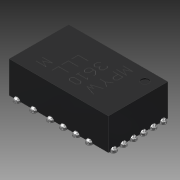
# Autodesk Inventor part: MPM3610 Step-Down Module
Saved by Autodesk Inventor 2016 (Build 200138000, 138)
## iProperties
Created: 2019-08-17
Part Number: MPM3610 Step-Down Module
Material: Generic
Document SubType Name: Modeling
Designer: Orest
Mass: 0.0242835 g
Surface Area: 0.598221 cm^2
Volume: 0.0242835 cm^3
Density: 1 g/cm^3
Appearance: Smooth - Black (BGA)
Author: Orest
Autodesk Inventor part; units mm, degrees
ref_plane "YZ Plane" through (0, 0, 0) normal (1, 0, 0) x (0, 1, 0)
ref_plane "XZ Plane" through (0, 0, 0) normal (0, 1, 0) x (-1, 0, 0)
sketch "Sketch10" plane through (0, 0, 0) normal (0, 1, 0) x (-1, 0, 0)
  line L0 (-1.5, -2.5) -> (1.5, -2.5)
  line L1 (1.5, -2.5) -> (1.5, 2.5)
  line L2 (1.5, 2.5) -> (-1.5, 2.5)
  line L3 (-1.5, 2.5) -> (-1.5, -2.5)
  line L4 (-1.5, -2.5) -> (1.5, 2.5) construction
  line L5 (1.5, -2.5) -> (-1.5, 2.5) construction
  point P0 (0, 0)
  point P1 (0, 0)
  dimension "d7" = 3
  dimension "d8" = 5
  constraints: 12 end point, 2 parallel, 1 coincident, 1 horizontal, 1 midpoint, 1 perpendicular
  measures "d7" distance of L1.end L2.end
  measures "d8" distance of L0.end L1.end
extrude "Extrusion4" add sketch "Sketch10" along normal mid plane 1.6
sketch "Sketch11" plane through (0, 0.8, 0) normal (0, 1, 0) x (1, 0, 0)
  circle A0 centre (0.95, -1.9) radius 0.2
  line L0 (1.5, 2.5) -> (-1.5, 2.5) construction
  line L1 (-1.5, 2.5) -> (-1.5, -2.5) construction
  line L2 (-1.5, -2.5) -> (1.5, -2.5) construction
  line L3 (1.5, -2.5) -> (1.5, 2.5) construction
  line L4 (1, -1.55) -> (-1, -1.55) construction
  line L5 (-1, -1.55) -> (-1, 2.1) construction
  line L6 (-1, 2.1) -> (1, 2.1) construction
  line L7 (1, 2.1) -> (1, -1.55) construction
  line L8 (0.7272, -0.6725) -> (0.7519, -0.6725)
  line L9 (0.7519, -0.6725) -> (0.7519, -1.1357)
  line L10 (0.7519, -1.1357) -> (0.9018, -0.8225)
  line L11 (0.9018, -0.8225) -> (1.0514, -1.1357)
  line L12 (1.0514, -1.1357) -> (1.0514, -0.6725)
  line L13 (1.0514, -0.6725) -> (1.076, -0.6725)
  line L14 (1.076, -0.6725) -> (1.076, -1.1725)
  line L15 (1.076, -1.1725) -> (1.0535, -1.1725)
  line L16 (1.0535, -1.1725) -> (0.9018, -0.8605)
  line L17 (0.9018, -0.8605) -> (0.7502, -1.1725)
  line L18 (0.7502, -1.1725) -> (0.7272, -1.1725)
  line L19 (0.7272, -1.1725) -> (0.7272, -0.6725)
  line L20 (0.2306, -0.9987) -> (0.3191, -0.9102)
  line L21 (0.3191, -0.9102) -> (0.5547, -0.9102)
  line L22 (0.5547, -0.9102) -> (0.5547, -0.6725)
  line L23 (0.5547, -0.6725) -> (0.5794, -0.6725)
  line L24 (0.5794, -0.6725) -> (0.5794, -1.1775)
  line L25 (0.5794, -1.1775) -> (0.3191, -1.1775)
  line L26 (0.3191, -1.1775) -> (0.2306, -1.089)
  line L27 (0.2306, -1.089) -> (0.2306, -0.9987)
  line L28 (0.2552, -1.0083) -> (0.2552, -1.0798)
  line L29 (0.2552, -1.0798) -> (0.3296, -1.1537)
  line L30 (0.3296, -1.1537) -> (0.5547, -1.1537)
  line L31 (0.5547, -1.1537) -> (0.5547, -0.9344)
  line L32 (0.5547, -0.9344) -> (0.3292, -0.9344)
  line L33 (0.3292, -0.9344) -> (0.2552, -1.0083)
  line L34 (-0.2652, -1.1654) -> (-0.1036, -0.9194)
  line L35 (-0.1036, -0.9194) -> (-0.1036, -0.6725)
  line L36 (-0.1036, -0.6725) -> (-0.0789, -0.6725)
  line L37 (-0.0789, -0.6725) -> (-0.0789, -0.9189)
  line L38 (-0.0789, -0.9189) -> (0.0823, -1.1654)
  line L39 (0.0823, -1.1654) -> (0.0639, -1.175)
  line L40 (0.0639, -1.175) -> (-0.0915, -0.9386)
  line L41 (-0.0915, -0.9386) -> (-0.2464, -1.175)
  line L42 (-0.2464, -1.175) -> (-0.2652, -1.1654)
  line L43 (-0.9244, -1.1675) -> (-0.7607, -0.6725)
  line L44 (-0.7607, -0.6725) -> (-0.7393, -0.6725)
  line L45 (-0.7393, -0.6725) -> (-0.6692, -0.8989)
  line L46 (-0.6692, -0.8989) -> (-0.5986, -0.6725)
  line L47 (-0.5986, -0.6725) -> (-0.5777, -0.6725)
  line L48 (-0.5777, -0.6725) -> (-0.414, -1.1675)
  line L49 (-0.414, -1.1675) -> (-0.4357, -1.1742)
  line L50 (-0.4357, -1.1742) -> (-0.5881, -0.703)
  line L51 (-0.5881, -0.703) -> (-0.6688, -0.9461)
  line L52 (-0.6688, -0.9461) -> (-0.7502, -0.703)
  line L53 (-0.7502, -0.703) -> (-0.9023, -1.1742)
  line L54 (-0.9023, -1.1742) -> (-0.9244, -1.1675)
  line L55 (0.3137, 0.0444) -> (0.4023, 0.1325)
  line L56 (0.4023, 0.1325) -> (0.5744, 0.1325)
  line L57 (0.5744, 0.1325) -> (0.6612, 0.0435)
  line L58 (0.6612, 0.0435) -> (0.6466, 0.0289)
  line L59 (0.6466, 0.0289) -> (0.5647, 0.1087)
  line L60 (0.5647, 0.1087) -> (0.4123, 0.1087)
  line L61 (0.4123, 0.1087) -> (0.3383, 0.0348)
  line L62 (0.3383, 0.0348) -> (0.3383, -0.0367)
  line L63 (0.3383, -0.0367) -> (0.4127, -0.1102)
  line L64 (0.4127, -0.1102) -> (0.495, -0.1102)
  line L65 (0.495, -0.1102) -> (0.495, -0.1344)
  line L66 (0.495, -0.1344) -> (0.4123, -0.1344)
  line L67 (0.4123, -0.1344) -> (0.3383, -0.2083)
  line L68 (0.3383, -0.2083) -> (0.3383, -0.2793)
  line L69 (0.3383, -0.2793) -> (0.4127, -0.3537)
  line L70 (0.4127, -0.3537) -> (0.5643, -0.3537)
  line L71 (0.5643, -0.3537) -> (0.6466, -0.2739)
  line L72 (0.6466, -0.2739) -> (0.6612, -0.2885)
  line L73 (0.6612, -0.2885) -> (0.5744, -0.3775)
  line L74 (0.5744, -0.3775) -> (0.4023, -0.3775)
  line L75 (0.4023, -0.3775) -> (0.3137, -0.289)
  line L76 (0.3137, -0.289) -> (0.3137, -0.1987)
  line L77 (0.3137, -0.1987) -> (0.3931, -0.1223)
  line L78 (0.3931, -0.1223) -> (0.3137, -0.0458)
  line L79 (0.3137, -0.0458) -> (0.3137, 0.0444)
  line L80 (-0.183, 0.0444) -> (-0.0944, 0.1325)
  line L81 (-0.0944, 0.1325) -> (0.0777, 0.1325)
  line L82 (0.0777, 0.1325) -> (0.1658, 0.0448)
  line L83 (0.1658, 0.0448) -> (0.1658, -0.2083)
  line L84 (0.1658, -0.2083) -> (-0.0033, -0.3775)
  line L85 (-0.0033, -0.3775) -> (-0.0961, -0.3775)
  line L86 (-0.0961, -0.3775) -> (-0.0961, -0.3537)
  line L87 (-0.0961, -0.3537) -> (-0.0134, -0.3537)
  line L88 (-0.0134, -0.3537) -> (0.1412, -0.1987)
  line L89 (0.1412, -0.1987) -> (0.1412, -0.1344)
  line L90 (0.1412, -0.1344) -> (-0.0944, -0.1344)
  line L91 (-0.0944, -0.1344) -> (-0.183, -0.0458)
  line L92 (-0.183, -0.0458) -> (-0.183, 0.0444)
  line L93 (-0.1583, 0.0348) -> (-0.1583, -0.0367)
  line L94 (-0.1583, -0.0367) -> (-0.084, -0.1102)
  line L95 (-0.084, -0.1102) -> (0.1412, -0.1102)
  line L96 (0.1412, -0.1102) -> (0.1412, 0.0352)
  line L97 (0.1412, 0.0352) -> (0.0681, 0.1087)
  line L98 (0.0681, 0.1087) -> (-0.0844, 0.1087)
  line L99 (-0.0844, 0.1087) -> (-0.1583, 0.0348)
  line L100 (-0.5121, 0.1325) -> (-0.3358, 0.1325)
  line L101 (-0.3358, 0.1325) -> (-0.3358, 0.1087)
  line L102 (-0.3358, 0.1087) -> (-0.4119, 0.1087)
  line L103 (-0.4119, 0.1087) -> (-0.4119, -0.3462)
  line L104 (-0.4119, -0.3462) -> (-0.3467, -0.2739)
  line L105 (-0.3467, -0.2739) -> (-0.3321, -0.2885)
  line L106 (-0.3321, -0.2885) -> (-0.4185, -0.3775)
  line L107 (-0.4185, -0.3775) -> (-0.4361, -0.3775)
  line L108 (-0.4361, -0.3775) -> (-0.4361, 0.1087)
  line L109 (-0.4361, 0.1087) -> (-0.5121, 0.1087)
  line L110 (-0.5121, 0.1087) -> (-0.5121, 0.1325)
  line L111 (-0.9298, 0.0444) -> (-0.8413, 0.1325)
  line L112 (-0.8413, 0.1325) -> (-0.7502, 0.1325)
  line L113 (-0.7502, 0.1325) -> (-0.6621, 0.0448)
  line L114 (-0.6621, 0.0448) -> (-0.6621, -0.2894)
  line L115 (-0.6621, -0.2894) -> (-0.7502, -0.3775)
  line L116 (-0.7502, -0.3775) -> (-0.8413, -0.3775)
  line L117 (-0.8413, -0.3775) -> (-0.9298, -0.289)
  line L118 (-0.9298, -0.289) -> (-0.9298, 0.0444)
  line L119 (-0.9052, 0.0348) -> (-0.9052, -0.2798)
  line L120 (-0.9052, -0.2798) -> (-0.8312, -0.3537)
  line L121 (-0.8312, -0.3537) -> (-0.7602, -0.3537)
  line L122 (-0.7602, -0.3537) -> (-0.6867, -0.2798)
  line L123 (-0.6867, -0.2798) -> (-0.6867, 0.0352)
  line L124 (-0.6867, 0.0352) -> (-0.7598, 0.1087)
  line L125 (-0.7598, 0.1087) -> (-0.8312, 0.1087)
  line L126 (-0.8312, 0.1087) -> (-0.9052, 0.0348)
  line L127 (0.071, 0.9325) -> (0.414, 0.9325)
  line L128 (0.414, 0.9325) -> (0.414, 0.4275)
  line L129 (0.414, 0.4275) -> (0.3893, 0.4275)
  line L130 (0.3893, 0.4275) -> (0.3893, 0.9087)
  line L131 (0.3893, 0.9087) -> (0.071, 0.9087)
  line L132 (0.071, 0.9087) -> (0.071, 0.9325)
  line L133 (-0.4256, 0.9325) -> (-0.0827, 0.9325)
  line L134 (-0.0827, 0.9325) -> (-0.0827, 0.4275)
  line L135 (-0.0827, 0.4275) -> (-0.1074, 0.4275)
  line L136 (-0.1074, 0.4275) -> (-0.1074, 0.9087)
  line L137 (-0.1074, 0.9087) -> (-0.4256, 0.9087)
  line L138 (-0.4256, 0.9087) -> (-0.4256, 0.9325)
  line L139 (-0.9223, 0.9325) -> (-0.5794, 0.9325)
  line L140 (-0.5794, 0.9325) -> (-0.5794, 0.4275)
  line L141 (-0.5794, 0.4275) -> (-0.604, 0.4275)
  line L142 (-0.604, 0.4275) -> (-0.604, 0.9087)
  line L143 (-0.604, 0.9087) -> (-0.9223, 0.9087)
  line L144 (-0.9223, 0.9087) -> (-0.9223, 0.9325)
  line L145 (-0.9282, 1.7275) -> (-0.9035, 1.7275)
  line L146 (-0.9035, 1.7275) -> (-0.9035, 1.2643)
  line L147 (-0.9035, 1.2643) -> (-0.7536, 1.5775)
  line L148 (-0.7536, 1.5775) -> (-0.604, 1.2643)
  line L149 (-0.604, 1.2643) -> (-0.604, 1.7275)
  line L150 (-0.604, 1.7275) -> (-0.5794, 1.7275)
  line L151 (-0.5794, 1.7275) -> (-0.5794, 1.2275)
  line L152 (-0.5794, 1.2275) -> (-0.6019, 1.2275)
  line L153 (-0.6019, 1.2275) -> (-0.7536, 1.5395)
  line L154 (-0.7536, 1.5395) -> (-0.9052, 1.2275)
  line L155 (-0.9052, 1.2275) -> (-0.9282, 1.2275)
  line L156 (-0.9282, 1.2275) -> (-0.9282, 1.7275)
  point P0 (0, 0)
  point P1 (0, -1.55)
  dimension "d11" = 0.4
  dimension "d12" = 0.4
  dimension "d13" = 3.65
  dimension "d14" = 2
  dimension "d15" = 0.6
  dimension "d16" = 0.55
  constraints: 1 centre point, 1 midpoint, 1 vertical alignment, 2 other
  measures "d11" diameter of A0
  measures "d12" distance between parallel lines of L0 L6
  measures "d13" distance between parallel lines of L4 L6
  measures "d14" distance between parallel lines of L7 L5
  measures "d15" distance from line of L2 A0.centre
  measures "d16" distance from line of L3 A0.centre
extrude "Extrusion5" cut sketch "Sketch11" against normal blind 0.01 contours L8 L9 L10 L11 L12 L13 L14 L15 L16 L17 L18 L19 | L20 L21 L22 L23 L24 L25 L26 L27 | L34 L35 L36 L37 L38 L39 L40 L41 L42 | L43 L44 L45 L46 L47 L48 L49 L50 L51 L52 L53 L54 | L55 L56 L57 L58 L59 L60 L61 L62 L63 L64 L65 L66 L67 L68 L69 L70 L71 L72 L73 L74 L75 L76 L77 L78 L79 | L80 L81 L82 L83 L84 L85 L86 L87 L88 L89 L90 L91 L92 | L100 L101 L102 L103 L104 L105 L106 L107 L108 L109 L110 | L111 L112 L113 L114 L115 L116 L117 L118 | L127 L128 L129 L130 L131 L132 | L133 L134 L135 L136 L137 L138 | L139 L140 L141 L142 L143 L144 | L145 L146 L147 L148 L149 L150 L151 L152 L153 L154 L155 L156
extrude "Extrusion6" cut sketch "Sketch11" against normal blind 0.075 contours A0
ref_plane "Work Plane1" through (0, -0.85, 0) normal (0, -1, 0) x (1, 0, 0)
sketch "Sketch12" plane through (0, -0.85, 0) normal (0, -1, 0) x (1, 0, 0)
  line L0 (-1.4, 2.65) -> (-1.1, 2.65)
  line L1 (-1.1, 2.65) -> (-1.1, 2.15)
  line L2 (-1.2, 2.05) -> (-1.3, 2.05)
  line L3 (-1.4, 2.15) -> (-1.4, 2.65)
  line L4 (-0.9, 2.65) -> (-0.6, 2.65)
  line L5 (-0.6, 2.65) -> (-0.6, 2.15)
  line L6 (-0.7, 2.05) -> (-0.8, 2.05)
  line L7 (-0.9, 2.15) -> (-0.9, 2.65)
  line L8 (-0.4, 2.65) -> (-0.1, 2.65)
  line L9 (-0.1, 2.65) -> (-0.1, 1.75)
  line L10 (-0.2, 1.65) -> (-0.3, 1.65)
  line L11 (-0.4, 1.75) -> (-0.4, 2.65)
  line L12 (-1.65, 1.05) -> (-0.75, 1.05)
  line L13 (-0.65, 0.95) -> (-0.65, 0.85)
  line L14 (-0.75, 0.75) -> (-1.65, 0.75)
  line L15 (-1.65, 0.75) -> (-1.65, 1.05)
  line L16 (-1.65, 0.4) -> (-0.75, 0.4)
  line L17 (-0.65, 0.3) -> (-0.65, 0.2)
  line L18 (-0.75, 0.1) -> (-1.65, 0.1)
  line L19 (-1.65, 0.1) -> (-1.65, 0.4)
  line L20 (-1.65, -0.25) -> (-0.75, -0.25)
  line L21 (-1.3, -0.55) -> (-1.65, -0.55)
  line L22 (-1.65, -0.55) -> (-1.65, -0.25)
  line L23 (-1.65, -1.1) -> (-1.3, -1.1)
  line L24 (-1.3, -1.4) -> (-1.65, -1.4)
  line L25 (-1.65, -1.4) -> (-1.65, -1.1)
  line L26 (-1.65, -1.95) -> (-1.3, -1.95)
  line L27 (-0.75, -2.25) -> (-1.65, -2.25)
  line L28 (-1.65, -2.25) -> (-1.65, -1.95)
  line L29 (-0.65, -0.35) -> (-0.65, -2.15)
  line L30 (-1.3, -1.1) -> (-1.3, -0.55)
  line L31 (-1.3, -1.95) -> (-1.3, -1.4)
  line L32 (-1.5, -2.5) -> (1.5, -2.5) construction
  line L33 (1.5, -2.5) -> (1.5, 2.5) construction
  line L34 (1.5, 2.5) -> (-1.5, 2.5) construction
  line L35 (-1.5, 2.5) -> (-1.5, -2.5) construction
  line L36 (-1.65, 1.4) -> (-1.15, 1.4)
  line L37 (-1.05, 1.5) -> (-1.05, 1.6)
  line L38 (-1.15, 1.7) -> (-1.65, 1.7)
  line L39 (-1.65, 1.7) -> (-1.65, 1.4)
  line L40 (0, 2.5) -> (0, -2.5) construction
  arc A0 (-0.75, -2.25) -> (-0.65, -2.15) centre (-0.75, -2.15) ccw
  arc A1 (-0.65, -0.35) -> (-0.75, -0.25) centre (-0.75, -0.35) ccw
  arc A2 (-0.75, 0.1) -> (-0.65, 0.2) centre (-0.75, 0.2) ccw
  arc A3 (-0.65, 0.3) -> (-0.75, 0.4) centre (-0.75, 0.3) ccw
  arc A4 (-0.75, 0.75) -> (-0.65, 0.85) centre (-0.75, 0.85) ccw
  arc A5 (-0.65, 0.95) -> (-0.75, 1.05) centre (-0.75, 0.95) ccw
  arc A6 (-1.15, 1.4) -> (-1.05, 1.5) centre (-1.15, 1.5) ccw
  arc A7 (-1.05, 1.6) -> (-1.15, 1.7) centre (-1.15, 1.6) ccw
  arc A8 (-1.4, 2.15) -> (-1.3, 2.05) centre (-1.3, 2.15) ccw
  arc A9 (-1.2, 2.05) -> (-1.1, 2.15) centre (-1.2, 2.15) ccw
  arc A10 (-0.9, 2.15) -> (-0.8, 2.05) centre (-0.8, 2.15) ccw
  arc A11 (-0.7, 2.05) -> (-0.6, 2.15) centre (-0.7, 2.15) ccw
  arc A12 (-0.4, 1.75) -> (-0.3, 1.65) centre (-0.3, 1.75) ccw
  arc A13 (-0.2, 1.65) -> (-0.1, 1.75) centre (-0.2, 1.75) ccw
  line L41 (1.4, 2.65) -> (1.1, 2.65)
  line L42 (1.1, 2.65) -> (1.1, 2.15)
  line L43 (1.2, 2.05) -> (1.3, 2.05)
  line L44 (1.4, 2.15) -> (1.4, 2.65)
  line L45 (0.9, 2.65) -> (0.6, 2.65)
  line L46 (0.6, 2.65) -> (0.6, 2.15)
  line L47 (0.7, 2.05) -> (0.8, 2.05)
  line L48 (0.9, 2.15) -> (0.9, 2.65)
  line L49 (0.4, 2.65) -> (0.1, 2.65)
  line L50 (0.1, 2.65) -> (0.1, 1.75)
  line L51 (0.2, 1.65) -> (0.3, 1.65)
  line L52 (0.4, 1.75) -> (0.4, 2.65)
  arc A14 (1.3, 2.05) -> (1.4, 2.15) centre (1.3, 2.15) ccw
  arc A15 (1.1, 2.15) -> (1.2, 2.05) centre (1.2, 2.15) ccw
  arc A16 (0.8, 2.05) -> (0.9, 2.15) centre (0.8, 2.15) ccw
  arc A17 (0.6, 2.15) -> (0.7, 2.05) centre (0.7, 2.15) ccw
  arc A18 (0.3, 1.65) -> (0.4, 1.75) centre (0.3, 1.75) ccw
  arc A19 (0.1, 1.75) -> (0.2, 1.65) centre (0.2, 1.75) ccw
  line L53 (1.65, 1.05) -> (0.75, 1.05)
  line L54 (0.65, 0.95) -> (0.65, 0.85)
  line L55 (0.75, 0.75) -> (1.65, 0.75)
  line L56 (1.65, 0.75) -> (1.65, 1.05)
  line L57 (1.65, 0.4) -> (0.75, 0.4)
  line L58 (0.65, 0.3) -> (0.65, 0.2)
  line L59 (0.75, 0.1) -> (1.65, 0.1)
  line L60 (1.65, 0.1) -> (1.65, 0.4)
  line L61 (1.65, -0.25) -> (0.75, -0.25)
  line L62 (1.3, -0.55) -> (1.65, -0.55)
  line L63 (1.65, -0.55) -> (1.65, -0.25)
  line L64 (1.65, -1.1) -> (1.3, -1.1)
  line L65 (1.3, -1.4) -> (1.65, -1.4)
  line L66 (1.65, -1.4) -> (1.65, -1.1)
  line L67 (1.65, -1.95) -> (1.3, -1.95)
  line L68 (0.75, -2.25) -> (1.65, -2.25)
  line L69 (1.65, -2.25) -> (1.65, -1.95)
  line L70 (0.65, -0.35) -> (0.65, -2.15)
  line L71 (1.3, -1.1) -> (1.3, -0.55)
  line L72 (1.3, -1.95) -> (1.3, -1.4)
  line L73 (1.65, 1.4) -> (1.15, 1.4) construction
  line L74 (1.05, 1.5) -> (1.05, 1.6) construction
  line L75 (1.15, 1.7) -> (1.65, 1.7) construction
  line L76 (1.65, 1.7) -> (1.65, 1.4) construction
  arc A20 (0.65, -2.15) -> (0.75, -2.25) centre (0.75, -2.15) ccw
  arc A21 (0.75, -0.25) -> (0.65, -0.35) centre (0.75, -0.35) ccw
  arc A22 (0.65, 0.2) -> (0.75, 0.1) centre (0.75, 0.2) ccw
  arc A23 (0.75, 0.4) -> (0.65, 0.3) centre (0.75, 0.3) ccw
  arc A24 (0.65, 0.85) -> (0.75, 0.75) centre (0.75, 0.85) ccw
  arc A25 (0.75, 1.05) -> (0.65, 0.95) centre (0.75, 0.95) ccw
  arc A26 (1.05, 1.5) -> (1.15, 1.4) centre (1.15, 1.5) ccw construction
  arc A27 (1.15, 1.7) -> (1.05, 1.6) centre (1.15, 1.6) ccw construction
  line L77 (1.65, 1.7) -> (1.075, 1.7)
  line L78 (0.95, 1.575) -> (0.95, 1.4)
  line L79 (0.95, 1.4) -> (1.65, 1.4)
  line L80 (1.65, 1.4) -> (1.65, 1.7)
  line L81 (0.95, 1.575) -> (1.075, 1.7)
  point P0 (0, 0)
  point P1 (-1.65, -1.25)
  point P2 (-0.65, -1.25)
  point P3 (1.65, -1.25)
  point P4 (0.65, -1.25)
  point P5 (0.95, 1.7)
  dimension "d22" = 0.3
  dimension "d29" = 0.25
  dimension "d30" = 0.15
  dimension "d31" = 0.2
  dimension "d33" = 2
  dimension "d34" = 0.85
  dimension "d39" = 0.8
  dimension "d40" = 0.35
  dimension "d41" = 0.35
  dimension "d43" = 0.45
  dimension "d44" = 0.15
  dimension "d49" = 0.1
  dimension "d50" = 0.2
  dimension "d51" = 0.2
  dimension "d52" = 0.2
  dimension "d53" = 0.55
  dimension "d54" = 0.125
  dimension "d55" = 0.125
  constraints: 156 end point, 66 symmetric about line, 56 point on circle, 28 centre point, 28 tangent, 19 parallel, 13 equal radius, 12 collinear, 10 equal length, 10 horizontal, 7 perpendicular, 6 point on line, 4 midpoint, 1 horizontal alignment, 14 other
  measures "d22" distance between parallel lines of L24 L23
  measures "d29" distance between parallel lines of L32 L27
  measures "d30" distance between parallel lines of L35 L28
  measures "d31" distance between parallel lines of L35 L31
  measures "d33" distance between parallel lines of L20 L27
  measures "d34" distance between parallel lines of L29 L35
  measures "d39" distance between parallel lines of L34 L38
  measures "d40" distance between parallel lines of L12 L36
  measures "d41" distance between parallel lines of L16 L14
  measures "d43" distance between parallel lines of L35 L37
  measures "d44" distance between parallel lines of L0 L34
  measures "d49" radius of A0
  measures "d50" distance between parallel lines of L50 L9
  measures "d51" distance between parallel lines of L5 L11
  measures "d52" distance between parallel lines of L1 L7
  measures "d53" distance between parallel lines of L33 L78
  measures "d54" distance of L78.start point (0.95, 1.7)
  measures "d55" distance of L77.end point (0.95, 1.7)
extrude "Extrusion7" add sketch "Sketch12" against normal blind 0.2
sketch "Sketch13" plane through (0, -0.8, 0) normal (0, -1, 0) x (1, 0, 0)
  line L0 (-0.65, 0.95) -> (-0.65, 0.85) projected
  line L1 (0.65, 0.95) -> (0.65, 0.85) projected
  line L2 (-0.2, 1.65) -> (-0.3, 1.65) projected
  line L3 (0.2, 1.65) -> (0.3, 1.65) projected
  line L4 (-0.575, 0.97) -> (0.575, 0.97)
  line L5 (0.575, 0.97) -> (0.575, 0.18)
  line L6 (0.575, 0.18) -> (-0.575, 0.18)
  line L7 (-0.575, 0.18) -> (-0.575, 0.97)
  line L8 (-1.5, 2.5) -> (1.5, 2.5) projected
  line L9 (-0.3375, 0.325) -> (-0.2375, 0.325)
  line L10 (-0.1375, 0.425) -> (-0.1375, 0.725)
  line L11 (-0.2375, 0.825) -> (-0.3375, 0.825)
  line L12 (-0.4375, 0.725) -> (-0.4375, 0.425)
  line L13 (0.2375, 0.325) -> (0.3375, 0.325)
  line L14 (0.4375, 0.425) -> (0.4375, 0.725)
  line L15 (0.3375, 0.825) -> (0.2375, 0.825)
  line L16 (0.1375, 0.725) -> (0.1375, 0.425)
  line L17 (1.65, 0.4) -> (0.75, 0.4) projected
  line L18 (0.75, 0.75) -> (1.65, 0.75) projected
  line L19 (-0.75, 0.75) -> (-1.65, 0.75) projected
  line L20 (-1.65, 0.4) -> (-0.75, 0.4) projected
  line L21 (-1.65, 0.75) -> (-1.65, 1.05) projected
  line L22 (0, 0.97) -> (0, 0.18) construction
  line L23 (-0.575, 0.97) -> (0, 0.97) construction
  arc A0 (-0.3375, 0.825) -> (-0.4375, 0.725) centre (-0.3375, 0.725) ccw
  arc A1 (-0.1375, 0.725) -> (-0.2375, 0.825) centre (-0.2375, 0.725) ccw
  arc A2 (-0.2375, 0.325) -> (-0.1375, 0.425) centre (-0.2375, 0.425) ccw
  arc A3 (-0.4375, 0.425) -> (-0.3375, 0.325) centre (-0.3375, 0.425) ccw
  arc A4 (0.2375, 0.825) -> (0.1375, 0.725) centre (0.2375, 0.725) ccw
  arc A5 (0.4375, 0.725) -> (0.3375, 0.825) centre (0.3375, 0.725) ccw
  arc A6 (0.3375, 0.325) -> (0.4375, 0.425) centre (0.3375, 0.425) ccw
  arc A7 (0.1375, 0.425) -> (0.2375, 0.325) centre (0.2375, 0.425) ccw
  line L24 (-0.4375, 0.575) -> (-0.1375, 0.575) construction
  point P0 (0, 0)
  point P1 (0, 2.5)
  point P2 (-0.2875, 0.97)
  point P3 (-0.2875, 0.825)
  point P4 (-0.575, 0.575)
  dimension "d60" = 1.15
  dimension "d61" = 1.53
  dimension "d62" = 0.79
  dimension "d63" = 0.5
  dimension "d64" = 0.1
  constraints: 30 end point, 16 point on circle, 16 tangent, 8 centre point, 8 midpoint, 7 equal radius, 6 parallel, 3 equal length, 3 horizontal, 3 perpendicular, 2 collinear, 2 vertical alignment, 1 horizontal alignment, 1 other
  measures "d60" distance between parallel lines of L5 L7
  measures "d61" distance between parallel lines of L8 L4
  measures "d62" distance between parallel lines of L6 L4
  measures "d63" distance between parallel lines of L9 L11
  measures "d64" radius of A0
extrude "Extrusion8" cut sketch "Sketch13" against normal blind 0.1
fillet "Fillet1" radius 0.15 90 edges at (1.65, -0.75, 1.7) (1.65, -0.75, 1.4) (1.65, -0.65, 1.55) (1.575, -0.65, 1.4) (1.575, -0.65, 1.7) (1.65, -0.75, 1.05) (1.65, -0.75, 0.75) (1.575, -0.65, 0.75) (1.65, -0.65, 0.9) (1.575, -0.65, 1.05) (1.65, -0.75, 0.4) (1.65, -0.75, 0.1) (1.65, -0.65, 0.25) (1.575, -0.65, 0.1) (1.575, -0.65, 0.4) (1.65, -0.75, -0.25) (1.65, -0.65, -0.4) (1.65, -0.75, -0.55) (1.575, -0.65, -0.55) (1.575, -0.65, -0.25) (1.65, -0.75, -1.4) (1.65, -0.65, -1.25) (1.65, -0.75, -1.1) (1.575, -0.65, -1.1) (1.575, -0.65, -1.4) (1.65, -0.75, -2.25) (1.65, -0.65, -2.1) (1.65, -0.75, -1.95) (1.575, -0.65, -1.95) (1.575, -0.65, -2.25) (1.4, -0.75, 2.65) (1.25, -0.65, 2.65) (1.1, -0.75, 2.65) (1.1, -0.65, 2.575) (1.4, -0.65, 2.575) (0.9, -0.75, 2.65) (0.75, -0.65, 2.65) (0.6, -0.75, 2.65) (0.6, -0.65, 2.575) (0.9, -0.65, 2.575) (0.4, -0.75, 2.65) (0.25, -0.65, 2.65) (0.1, -0.75, 2.65) (0.1, -0.65, 2.575) (0.4, -0.65, 2.575) (-0.1, -0.75, 2.65) (-0.25, -0.65, 2.65) (-0.4, -0.75, 2.65) (-0.4, -0.65, 2.575) (-0.1, -0.65, 2.575) (-0.6, -0.75, 2.65) (-0.75, -0.65, 2.65) (-0.9, -0.75, 2.65) (-0.9, -0.65, 2.575) (-0.6, -0.65, 2.575) (-1.1, -0.75, 2.65) (-1.25, -0.65, 2.65) (-1.4, -0.75, 2.65) (-1.4, -0.65, 2.575) (-1.1, -0.65, 2.575) (-1.65, -0.75, 1.7) (-1.65, -0.75, 1.4) (-1.65, -0.75, 1.05) (-1.65, -0.75, 0.75) (-1.65, -0.75, 0.4) (-1.65, -0.75, 0.1) (-1.65, -0.75, -0.25) (-1.65, -0.75, -0.55) (-1.65, -0.75, -1.1) (-1.65, -0.75, -1.4) (-1.65, -0.75, -1.95) (-1.65, -0.75, -2.25) (-1.65, -0.65, -2.1) (-1.575, -0.65, -2.25) (-1.575, -0.65, -1.95) (-1.65, -0.65, -1.25) (-1.575, -0.65, -1.4) (-1.575, -0.65, -1.1) (-1.65, -0.65, -0.4) (-1.575, -0.65, -0.55) (-1.575, -0.65, -0.25) (-1.65, -0.65, 0.25) (-1.575, -0.65, 0.1) (-1.575, -0.65, 0.4) (-1.65, -0.65, 0.9) (-1.575, -0.65, 0.75) (-1.575, -0.65, 1.05) (-1.65, -0.65, 1.55) (-1.575, -0.65, 1.4) (-1.575, -0.65, 1.7)
equation "\"d41\" = d40"
equation "\"d44\" = d30"
equation "\"d51\" = d50"
equation "\"d52\" = d51"
equation "\"d55\" = d54"
equation "\"d67\" = d30"
body "Solid4"
